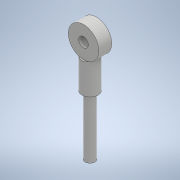
# Autodesk Inventor part: ダンパー下パーツ
Saved by Autodesk Inventor 2020.2 (Build 242310000, 310)
## iProperties
Created: 2018-03-29
Part Number: ダンパー下パーツ
Material: 一般
Document SubType Name: Modeling
Designer: Takumi
Density: 1 g/cm^3
Appearance: 既定
Mass: 0.570957 g
Surface Area: 6.13148 cm^2
Volume: 0.570957 cm^3
Author: Takumi
Autodesk Inventor part; units mm, degrees
ref_plane "YZ Plane" through (0, 0, 0) normal (1, 0, 0) x (0, 1, 0)
ref_plane "XZ Plane" through (0, 0, 0) normal (0, 1, 0) x (-1, 0, 0)
sketch "スケッチ1" plane through (0, 0, 0) normal (0, 0, 1) x (1, 0, 0)
  circle A0 centre (0, 0) radius 1.5
  circle A1 centre (0, 0) radius 2.5
  line L0 (0, 0) -> (0, 2.5)
  dimension "d1" = 5
  dimension "d0" = 3
  constraints: 2 coincident, 2 end point, 1 centre point, 1 vertical, 1 vertical alignment, 2 other
  measures "d0" diameter of A0
extrude "押し出し1" add sketch "スケッチ1" along normal blind 14 contours A0 | A1
extrude "押し出し2" add sketch "スケッチ1" against normal blind 18.5 contours A0
ref_plane "作業平面1" through (0, 0, 0) normal (0, 1, 0) x (-1, 0, 0)
sketch "スケッチ2" plane through (0, 0, 0) normal (0, 1, 0) x (-1, 0, 0)
  line L0 (2.5, 14) -> (-2.5, 14) projected
  circle A0 centre (0, 14) radius 4.75
  point P0 (0, 0)
  dimension "d6" = 9.5
  constraints: 1 centre point, 1 midpoint
  measures "d6" diameter of A0
extrude "押し出し3" add sketch "スケッチ2" along normal mid plane 4
sketch "スケッチ3" plane through (0, 2, 0) normal (0, 1, 0) x (1, 0, 0)
  line L0 (-1.5, -14) -> (1.5, -14) projected
  circle A0 centre (0, -14) radius 4.75
  point P0 (0, 0)
  dimension "d9" = 9.5
  constraints: 1 centre point, 1 midpoint
  measures "d9" diameter of A0
extrude "押し出し4" cut sketch "スケッチ3" along normal blind 4
sketch "スケッチ4" plane through (0, -2, 0) normal (0, -1, 0) x (1, 0, 0)
  line L0 (1.5, 14) -> (-1.5, 14) projected
  circle A0 centre (0, 14) radius 4.75
  point P0 (0, 0)
  dimension "d12" = 9.5
  constraints: 1 centre point, 1 midpoint
  measures "d12" diameter of A0
extrude "押し出し5" cut sketch "スケッチ4" along normal blind 4
hole "穴1" at (0, -2, 14) direction (0, 1, 0) diameter 3 end through all
sketch "スケッチ5" plane through (0, 0, 0) normal (0, 0, -1) x (-1, 0, 0)
  circle A0 centre (0, 0) radius 2.5 projected
  circle A1 centre (0, 0) radius 1.5 projected
